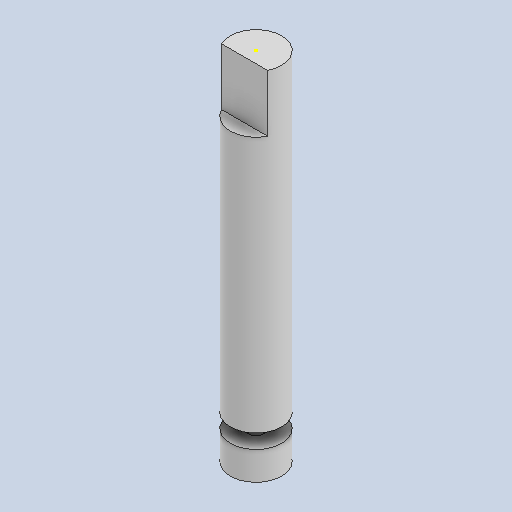
# Autodesk Inventor part: Деталь1
Saved by Autodesk Inventor 2022 (Build 260153000, 153)
## iProperties
Created: 2021-04-16
Part Number: Деталь1
Material: Типовые
Document SubType Name: Modeling
Designer: lbfas
Density: 1 g/cm^3
Appearance: По умолчанию
Author: lbfas
Autodesk Inventor part; units mm, degrees
ref_plane "YZ Plane" through (0, 0, 0) normal (1, 0, 0) x (0, 1, 0)
ref_plane "XZ Plane" through (0, 0, 0) normal (0, 1, 0) x (-1, 0, 0)
ref_plane "XY Plane" through (0, 0, 0) normal (0, 0, 1) x (1, 0, 0)
sketch "Эскиз1" plane through (0, 0, 0) normal (0, 1, 0) x (-1, 0, 0)
  circle A0 centre (0, 0) radius 4.5
  dimension "d0" = 9
  constraints: 1 centre point, 1 coincident
  measures "d0" diameter of A0
sketch "Эскиз5" plane through (0, 0, 0) normal (0, 1, 0) x (-1, 0, 0)
  point P0 (0, 0)
extrude "Выдавливание4" add sketch "Эскиз1" along normal blind 5
sketch "Эскиз6" plane through (0, 5, 0) normal (0, 1, 0) x (1, 0, 0)
  circle A0 centre (0, 0) radius 4.5 projected
  circle A1 centre (0, 0) radius 1.5
  dimension "d12" = 3
  constraints: 1 centre point, 1 coincident
  measures "d12" diameter of A1
extrude "Выдавливание5" add sketch "Эскиз6" along normal blind 2.5 contours A1
sketch "Эскиз7" plane through (0, 7.5, 0) normal (0, 1, 0) x (1, 0, 0)
  circle A0 centre (0, 0) radius 4.5
  dimension "d15" = 9
  constraints: 1 centre point, 1 coincident
  measures "d15" diameter of A0
extrude "Выдавливание6" add sketch "Эскиз7" along normal blind 55
sketch "Эскиз8" plane through (0, 62.5, 0) normal (0, 1, 0) x (1, 0, 0)
  line L0 (0, 0) -> (0, -2)
  line L1 (0, -2) -> (-5.0098, -2)
  line L2 (0, -2) -> (5.0098, -2)
  line L3 (5.0098, -2) -> (5.0098, -6.5905)
  line L4 (5.0098, -6.5905) -> (-5.0098, -6.5905)
  line L5 (-5.0098, -6.5905) -> (-5.0098, -2)
  dimension "d18" = 2
  constraints: 12 end point, 2 perpendicular, 2 vertical, 1 horizontal, 1 symmetric about line
  measures "d18" distance of L0.start L0.end
sketch "Эскиз9" plane through (0, 62.5, 0) normal (0, 1, 0) x (1, 0, 0)
  point P0 (0, 0)
extrude "Выдавливание7" cut sketch "Эскиз8" against normal blind 10
